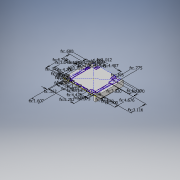
# Autodesk Inventor part: RioCoverPlate
Saved by Autodesk Inventor 2017 SP1 (Build 210196100, 196)
## iProperties
Created: 2016-11-23
Part Number: RioCoverPlate
Material: Generic
Document SubType Name: Modeling
Designer: steele
Density: 1 g/cm^3
Appearance: Default
Author: steele
Autodesk Inventor part; units mm, degrees
ref_plane "YZ Plane" through (0, 0, 0) normal (1, 0, 0) x (0, 1, 0)
ref_plane "XZ Plane" through (0, 0, 0) normal (0, 1, 0) x (-1, 0, 0)
ref_plane "XY Plane" through (0, 0, 0) normal (0, 0, 1) x (1, 0, 0)
sketch "Sketch1" plane through (0, 0, 0) normal (0, 0, 1) x (1, 0, 0)
  line L0 (0, 26.035) -> (-84.1883, 26.035)
  line L1 (-84.1883, 26.035) -> (-84.1883, 0)
  line L2 (-84.1883, 0) -> (-74.6633, 0)
  line L3 (-74.6633, 0) -> (-74.6633, 22.86)
  line L4 (-74.6633, 22.86) -> (0, 22.86)
  line L5 (0, 0) -> (0, 26.035) construction
  line L6 (0, 26.035) -> (84.1883, 26.035)
  line L7 (84.1883, 26.035) -> (84.1883, 0)
  line L8 (84.1883, 0) -> (74.6633, 0)
  line L9 (74.6633, 0) -> (74.6633, 22.86)
  line L10 (74.6633, 22.86) -> (0, 22.86)
  dimension "d0" = 22.86
  dimension "d1" = 3.175
  dimension "d2" = 9.525
  dimension "d3" = 74.6633
  constraints: 22 end point, 4 perpendicular, 4 symmetric about line, 1 horizontal, 1 vertical
  measures "d0" distance from line of L4 L5.start
  measures "d1" distance between parallel lines of L0 L4
  measures "d2" distance of L1.end L2.end
  measures "d3" distance of L2.end L5.start
extrude "Extrusion1" add sketch "Sketch1" along normal mid plane 143.1798
sketch "Sketch2" plane through (-84.1883, 0, 71.5899) normal (0, -1, 0) x (1, 0, 0)
  line L0 (0, -143.1798) -> (168.3766, -143.1798) construction
  line L1 (4.7625, -143.1798) -> (4.7625, -0.1575) construction
  line L2 (0, 0) -> (9.525, 0) projected
  point P0 (84.1883, -71.5899)
  point P1 (4.7625, -117.7798)
  point P2 (4.7625, -25.4)
  dimension "d6" = 4.7625
  dimension "d7" = 25.4
  dimension "d8" = 25.4
  constraints: 3 point on line, 2 end point, 1 vertical
  measures "d6" distance of L0.start L1.start
  measures "d7" distance of point (4.763, -117.78) L1.start
  measures "d8" distance from line of point (4.763, -25.4) L2
hole "Hole1" at (-79.4258, 0, -46.1899) at (-79.4258, 0, 46.1899) direction (0, 1, 0) diameter 5.1054 end through all clearance for "Flat Head Machine Screw (82)" size "#10" standard "Ansi Unified Screw Threads"
mirror "Mirror1" about plane through (0, 0, 0) normal (1, 0, 0) of "Hole1"
sketch "Sketch3" plane through (-84.1883, 26.035, 71.5899) normal (0, 1, 0) x (1, 0, 0)
  line L0 (11.1125, 0) -> (157.2641, 0) construction
  line L1 (157.2641, 0) -> (157.2641, 143.1798) construction
  line L2 (157.2641, 143.1798) -> (11.1125, 143.1798) construction
  line L3 (11.1125, 143.1798) -> (11.1125, 0) construction
  line L4 (11.1125, 0) -> (157.2641, 143.1798) construction
  line L5 (157.2641, 0) -> (11.1125, 143.1798) construction
  line L6 (51.9303, 1.2954) -> (83.4263, 1.2954)
  line L7 (83.4263, 1.2954) -> (83.4263, 9.9314)
  line L8 (83.4263, 9.9314) -> (51.9303, 9.9314)
  line L9 (51.9303, 9.9314) -> (51.9303, 1.2954)
  line L10 (51.9303, 1.2954) -> (83.4263, 9.9314) construction
  line L11 (83.4263, 1.2954) -> (51.9303, 9.9314) construction
  line L12 (168.3766, 0) -> (0, 0) projected
  line L13 (84.9503, 1.2954) -> (116.4463, 1.2954)
  line L14 (116.4463, 1.2954) -> (116.4463, 9.9314)
  line L15 (116.4463, 9.9314) -> (84.9503, 9.9314)
  line L16 (84.9503, 9.9314) -> (84.9503, 1.2954)
  line L17 (84.9503, 1.2954) -> (116.4463, 9.9314) construction
  line L18 (116.4463, 1.2954) -> (84.9503, 9.9314) construction
  line L19 (123.5075, 2.8702) -> (145.4785, 2.8702)
  line L20 (145.4785, 2.8702) -> (145.4785, 20.6502)
  line L21 (145.4785, 20.6502) -> (123.5075, 20.6502)
  line L22 (123.5075, 20.6502) -> (123.5075, 2.8702)
  line L23 (123.5075, 2.8702) -> (145.4785, 20.6502) construction
  line L24 (145.4785, 2.8702) -> (123.5075, 20.6502) construction
  line L25 (15.2273, 15.1892) -> (24.7523, 15.1892)
  line L26 (24.7523, 15.1892) -> (24.7523, 92.4052)
  line L27 (24.7523, 92.4052) -> (15.2273, 92.4052)
  line L28 (15.2273, 92.4052) -> (15.2273, 15.1892)
  line L29 (15.2273, 15.1892) -> (24.7523, 92.4052) construction
  line L30 (24.7523, 15.1892) -> (15.2273, 92.4052) construction
  line L31 (123.0503, 118.7704) -> (133.0833, 118.7704)
  line L32 (133.0833, 118.7704) -> (133.0833, 140.8684)
  line L33 (133.0833, 140.8684) -> (123.0503, 140.8684)
  line L34 (123.0503, 140.8684) -> (123.0503, 118.7704)
  line L35 (123.0503, 118.7704) -> (133.0833, 140.8684) construction
  line L36 (133.0833, 118.7704) -> (123.0503, 140.8684) construction
  line L37 (137.5791, 97.028) -> (157.2641, 97.028)
  line L38 (157.2641, 97.028) -> (157.2641, 133.096)
  line L39 (157.2641, 133.096) -> (137.5791, 133.096)
  line L40 (137.5791, 133.096) -> (137.5791, 97.028)
  line L41 (137.5791, 97.028) -> (157.2641, 133.096) construction
  line L42 (157.2641, 97.028) -> (137.5791, 133.096) construction
  line L43 (144.5133, 16.3322) -> (154.0383, 16.3322)
  line L44 (154.0383, 16.3322) -> (154.0383, 95.4786)
  line L45 (154.0383, 95.4786) -> (144.5133, 95.4786)
  line L46 (144.5133, 95.4786) -> (144.5133, 16.3322)
  line L47 (144.5133, 16.3322) -> (154.0383, 95.4786) construction
  line L48 (154.0383, 16.3322) -> (144.5133, 95.4786) construction
  line L49 (36.8173, 121.8184) -> (48.1203, 121.8184)
  line L50 (48.1203, 121.8184) -> (48.1203, 139.0904)
  line L51 (48.1203, 139.0904) -> (36.8173, 139.0904)
  line L52 (36.8173, 139.0904) -> (36.8173, 121.8184)
  line L53 (36.8173, 121.8184) -> (48.1203, 139.0904) construction
  line L54 (48.1203, 121.8184) -> (36.8173, 139.0904) construction
  line L55 (29.0703, 4.1148) -> (37.8333, 4.1148)
  line L56 (37.8333, 4.1148) -> (37.8333, 12.8778)
  line L57 (37.8333, 12.8778) -> (29.0703, 12.8778)
  line L58 (29.0703, 12.8778) -> (29.0703, 4.1148)
  line L59 (29.0703, 4.1148) -> (37.8333, 12.8778) construction
  line L60 (37.8333, 4.1148) -> (29.0703, 12.8778) construction
  line L61 (15.2273, 95.2754) -> (24.7523, 95.2754)
  line L62 (24.7523, 95.2754) -> (24.7523, 104.8004)
  line L63 (24.7523, 104.8004) -> (15.2273, 104.8004)
  line L64 (15.2273, 104.8004) -> (15.2273, 95.2754)
  line L65 (15.2273, 95.2754) -> (24.7523, 104.8004) construction
  line L66 (24.7523, 95.2754) -> (15.2273, 104.8004) construction
  line L67 (15.2273, 106.68) -> (25.8953, 106.68)
  line L68 (25.8953, 106.68) -> (25.8953, 114.681)
  line L69 (25.8953, 114.681) -> (15.2273, 114.681)
  line L70 (15.2273, 114.681) -> (15.2273, 106.68)
  line L71 (15.2273, 106.68) -> (25.8953, 114.681) construction
  line L72 (25.8953, 106.68) -> (15.2273, 114.681) construction
  point P0 (84.1883, 71.5899)
  point P1 (67.6783, 5.6134)
  point P2 (100.6983, 5.6134)
  point P3 (134.493, 11.7602)
  point P4 (19.9898, 53.7972)
  point P5 (128.0668, 129.8194)
  point P6 (147.4216, 115.062)
  point P7 (149.2758, 55.9054)
  point P8 (42.4688, 130.4544)
  point P9 (33.4518, 8.4963)
  point P10 (19.9898, 100.0379)
  point P11 (20.5613, 110.6805)
  dimension "d16" = 143.1798
  dimension "d17" = 146.1516
  dimension "d18" = 31.496
  dimension "d19" = 8.636
  dimension "d20" = 40.8178
  dimension "d21" = 1.2954
  dimension "d22" = 31.496
  dimension "d23" = 8.636
  dimension "d24" = 73.8378
  dimension "d25" = 1.2954
  dimension "d26" = 17.78
  dimension "d27" = 21.971
  dimension "d28" = 2.8702
  dimension "d29" = 112.395
  dimension "d30" = 77.216
  dimension "d31" = 9.525
  dimension "d32" = 15.1892
  dimension "d33" = 4.1148
  dimension "d34" = 10.033
  dimension "d35" = 22.098
  dimension "d36" = 111.9378
  dimension "d37" = 118.7704
  dimension "d38" = 19.685
  dimension "d39" = 36.068
  dimension "d40" = 97.028
  dimension "d41" = 9.525
  dimension "d42" = 79.1464
  dimension "d43" = 16.3322
  dimension "d44" = 133.4008
  dimension "d45" = 11.303
  dimension "d46" = 17.272
  dimension "d47" = 25.7048
  dimension "d48" = 121.8184
  dimension "d49" = 8.763
  dimension "d50" = 8.763
  dimension "d51" = 17.9578
  dimension "d52" = 4.1148
  dimension "d53" = 9.525
  dimension "d54" = 9.525
  dimension "d55" = 95.2754
  dimension "d56" = 4.1148
  dimension "d57" = 10.668
  dimension "d58" = 8.001
  dimension "d59" = 4.1148
  dimension "d60" = 106.68
  constraints: 144 end point, 26 parallel, 24 midpoint, 14 perpendicular, 8 horizontal, 1 collinear
  measures "d16" distance of L2.end L0.start
  measures "d17" distance of L0.start L0.end
  measures "d18" distance of L6.start L6.end
  measures "d19" distance of L8.end L6.start
  measures "d20" distance between parallel lines of L3 L9
  measures "d21" distance between parallel lines of L0 L6
  measures "d22" distance of L13.start L13.end
  measures "d23" distance of L13.end L14.end
  measures "d24" distance between parallel lines of L16 L3
  measures "d25" distance between parallel lines of L12 L13
  measures "d26" distance of L19.end L20.end
  measures "d27" distance of L19.start L19.end
  measures "d28" distance between parallel lines of L19 L12
  measures "d29" distance between parallel lines of L22 L3
  measures "d30" distance of L27.end L25.start
  measures "d31" distance of L25.start L25.end
  measures "d32" distance between parallel lines of L25 L12
  measures "d33" distance between parallel lines of L3 L28
  measures "d34" distance of L32.end L33.end
  measures "d35" distance of L31.end L32.end
  measures "d36" distance between parallel lines of L34 L3
  measures "d37" distance between parallel lines of L0 L31
  measures "d38" distance of L38.end L39.end
  measures "d39" distance of L37.end L38.end
  measures "d40" distance between parallel lines of L12 L37
  measures "d41" distance of L43.start L43.end
  measures "d42" distance of L43.end L44.end
  measures "d43" distance between parallel lines of L43 L12
  measures "d44" distance between parallel lines of L46 L3
  measures "d45" distance of L50.end L51.end
  measures "d46" distance of L51.end L49.start
  measures "d47" distance between parallel lines of L52 L3
  measures "d48" distance between parallel lines of L0 L49
  measures "d49" distance of L55.start L55.end
  measures "d50" distance of L57.end L55.start
  measures "d51" distance between parallel lines of L58 L3
  measures "d52" distance between parallel lines of L55 L12
  measures "d53" distance of L62.end L63.end
  measures "d54" distance of L63.end L61.start
  measures "d55" distance between parallel lines of L61 L0
  measures "d56" distance between parallel lines of L3 L64
  measures "d57" distance of L68.end L69.end
  measures "d58" distance of L69.end L67.start
  measures "d59" distance between parallel lines of L3 L70
  measures "d60" distance between parallel lines of L0 L67
equation "\"d0\" = heightForRIO"
equation "\"d1\" = topWallThickness"
equation "\"d2\" = edgeWallThickness"
equation "\"d3\" = 0.5 * widthOfRIO + widthAirGap"
equation "\"d4\" = depthOfRIO"
equation "\"d6\" = 0.5 * edgeWallThickness"
equation "\"d16\" = depthOfRIO"
equation "\"d17\" = widthOfRIO"
equation "\"d18\" = widthForBottomRelay"
equation "\"d19\" = depthForBottomRelay"
equation "\"d20\" = edgeToBottomRelay"
equation "\"d21\" = bottomToBottomRelay"
equation "\"d22\" = widthForBottomAnalogIn"
equation "\"d23\" = depthForBottomAnalogIn"
equation "\"d24\" = edgeToBottomAnalogIn"
equation "\"d25\" = bottomToBottomAnalogIn"
equation "\"d26\" = buttonDepth"
equation "\"d27\" = buttonWidth"
equation "\"d28\" = bottomToBottomButton"
equation "\"d29\" = edgeToBottomButton"
equation "\"d30\" = depthLeftDIO"
equation "\"d31\" = widthLeftDIO"
equation "\"d32\" = bottomToLeftDIO"
equation "\"d33\" = edgeToLeftDIO"
equation "\"d34\" = widthSPI"
equation "\"d35\" = depthSPI"
equation "\"d36\" = edgeToSPI"
equation "\"d37\" = bottomToSPI"
equation "\"d38\" = widthLight"
equation "\"d39\" = depthLight"
equation "\"d40\" = bottomToLight"
equation "\"d41\" = widthPWM"
equation "\"d42\" = depthPWM"
equation "\"d43\" = bottomToPWM"
equation "\"d44\" = edgeToPWM"
equation "\"d45\" = widthPower"
equation "\"d46\" = depthPower"
equation "\"d47\" = edgeToPower"
equation "\"d48\" = bottomToPower"
equation "\"d49\" = widthRSL"
equation "\"d50\" = depthRSL"
equation "\"d51\" = edgeToRSL"
equation "\"d52\" = bottomToRSL"
equation "\"d53\" = widthRS232"
equation "\"d54\" = depthRS232"
equation "\"d55\" = bottomToRS232"
equation "\"d56\" = edgeToRS232"
equation "\"d57\" = widthI2C"
equation "\"d58\" = depthI2C"
equation "\"d59\" = edgeToI2C"
equation "\"d60\" = bottomToI2C"
equation "\"heightForRIO\" = 22.86"
equation "\"topWallThickness\" = 3.175"
equation "\"edgeWallThickness\" = 9.525"
equation "\"widthOfRIO\" = 146.1516"
equation "\"widthAirGap\" = 1.5875"
equation "\"depthOfRIO\" = 143.1798"
equation "\"depthForBottomRelay\" = 8.636"
equation "\"widthForBottomRelay\" = 31.496"
equation "\"componentGap\" = 3.175"
equation "\"edgeToBottomRelay\" = 40.8178"
equation "\"bottomToBottomRelay\" = 1.2954"
equation "\"depthForBottomAnalogIn\" = 8.636"
equation "\"widthForBottomAnalogIn\" = 31.496"
equation "\"edgeToBottomAnalogIn\" = 73.8378"
equation "\"bottomToBottomAnalogIn\" = 1.2954"
equation "\"buttonWidth\" = 21.971"
equation "\"buttonDepth\" = 17.78"
equation "\"bottomToBottomButton\" = 2.8702"
equation "\"edgeToBottomButton\" = 112.395"
equation "\"widthLeftDIO\" = 9.525"
equation "\"depthLeftDIO\" = 77.216"
equation "\"bottomToLeftDIO\" = 15.1892"
equation "\"edgeToLeftDIO\" = 4.1148"
equation "\"widthSPI\" = 10.033"
equation "\"depthSPI\" = 22.098"
equation "\"edgeToSPI\" = 111.9378"
equation "\"bottomToSPI\" = 118.7704"
equation "\"widthLight\" = 19.685"
equation "\"depthLight\" = 36.068"
equation "\"bottomToLight\" = 97.028"
equation "\"widthPWM\" = 9.525"
equation "\"depthPWM\" = 79.1464"
equation "\"bottomToPWM\" = 16.3322"
equation "\"edgeToPWM\" = 133.4008"
equation "\"widthPower\" = 11.303"
equation "\"depthPower\" = 17.272"
equation "\"edgeToPower\" = 25.7048"
equation "\"bottomToPower\" = 121.8184"
equation "\"widthRSL\" = 8.763"
equation "\"depthRSL\" = 8.763"
equation "\"bottomToRSL\" = 4.1148"
equation "\"edgeToRSL\" = 17.9578"
equation "\"widthRS232\" = 9.525"
equation "\"depthRS232\" = 9.525"
equation "\"bottomToRS232\" = 95.2754"
equation "\"edgeToRS232\" = 4.1148"
equation "\"widthI2C\" = 10.668"
equation "\"depthI2C\" = 8.001"
equation "\"edgeToI2C\" = 4.1148"
equation "\"bottomToI2C\" = 106.68"
body "Solid1"
